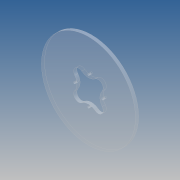
# Autodesk Inventor part: Plato T5
Saved by Autodesk Inventor 2017 (Build 210142000, 142)
## iProperties
Part Number: Plato T5
Material: Genérico
Document SubType Name: Modeling
Designer: Leo
Density: 1 g/cm^3
Appearance: Claro - Ligero
Author: Leo
Autodesk Inventor part; units mm, degrees
ref_plane "YZ Plane" through (0, 0, 0) normal (1, 0, 0) x (0, 1, 0)
ref_plane "XZ Plane" through (0, 0, 0) normal (0, 1, 0) x (-1, 0, 0)
ref_plane "XY Plane" through (0, 0, 0) normal (0, 0, 1) x (1, 0, 0)
sketch "Boceto1" plane through (0, 0, 0) normal (0, 1, 0) x (-1, 0, 0)
  circle A0 centre (0, 0) radius 15
  circle A1 centre (0, 0) radius 75
  arc A2 (-10.6675, 21.8887) -> (10.6675, 21.8887) centre (0, 35.706) ccw projected
  arc A3 (21.8887, 10.6675) -> (10.6675, 21.8887) centre (15.5563, 15.5563) ccw projected
  arc A4 (21.8887, 10.6675) -> (21.8887, -10.6675) centre (35.706, 0) ccw projected
  arc A5 (10.6675, -21.8887) -> (21.8887, -10.6675) centre (15.5563, -15.5563) ccw projected
  arc A6 (10.6675, -21.8887) -> (-10.6675, -21.8887) centre (0, -35.706) ccw projected
  arc A7 (-21.8887, -10.6675) -> (-10.6675, -21.8887) centre (-15.5563, -15.5563) ccw projected
  arc A8 (-21.8887, -10.6675) -> (-21.8887, 10.6675) centre (-35.706, 0) ccw projected
  arc A9 (-10.6675, 21.8887) -> (-21.8887, 10.6675) centre (-15.5563, 15.5563) ccw projected
  circle A10 centre (0, -22.5) radius 1.5 projected
  circle A11 centre (22.5, 0) radius 1.5 projected
  circle A12 centre (0, 22.5) radius 1.5 projected
  circle A13 centre (-22.5, 0) radius 1.5 projected
  circle A14 centre (0, 0) radius 15.25 projected
  dimension "d0" = 30
  dimension "d1" = 150
  constraints: 2 centre point, 2 coincident
  measures "d0" diameter of A0
  measures "d1" diameter of A1
extrude "Extrusión1" add sketch "Boceto1" along normal blind 5 contours A1
